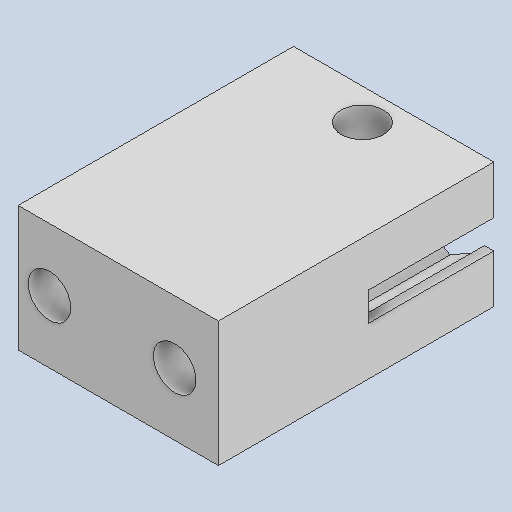
# Autodesk Inventor part: belt_holder
Saved by Autodesk Inventor 2024 (Build 280153000, 153)
## iProperties
Created: 2026-02-15
Part Number: belt_holder
Material: Generic
Document SubType Name: Modeling
Designer: SEMEN
Density: 1 g/cm^3
Appearance: Default
Author: SEMEN
Autodesk Inventor part; units mm, degrees
ref_plane "YZ Plane" through (0, 0, 0) normal (1, 0, 0) x (0, 1, 0)
ref_plane "XZ Plane" through (0, 0, 0) normal (0, 1, 0) x (-1, 0, 0)
sketch "Sketch1" plane through (0, 0, 0) normal (0, 0, 1) x (1, 0, 0)
  circle A0 centre (-12.704, 28.2207) radius 12 projected
  circle A1 centre (-12.704, -22.5861) radius 12 projected
  line L0 (-12.704, 28.2207) -> (-12.704, -22.5861) construction
  line L1 (4.1406, 2.8173) -> (-27.9996, 2.8173) construction
  line L2 (-24.704, -73.8176) -> (-24.704, 176.1824) projected
  line L3 (-5.204, -22.5861) -> (-5.204, 28.2207) projected
  line L4 (-22.204, -2.1827) -> (-6.204, -2.1827)
  line L5 (-6.204, -2.1827) -> (-6.204, 7.8173)
  line L6 (-6.204, 7.8173) -> (-22.204, 7.8173)
  line L7 (-22.204, 7.8173) -> (-22.204, -2.1827)
  circle A2 centre (-9.704, 2.8173) radius 3.5 construction
  circle A3 centre (-19.704, 2.8173) radius 2.5 construction
  point P0 (0, 0)
  point P1 (-12.704, 2.8173)
  dimension "d1" = 10
  dimension "d2" = 5
  dimension "d3" = 7
  dimension "d4" = 5
  dimension "d5" = 10
  constraints: 12 end point, 3 point on line, 2 centre point, 2 coincident, 2 horizontal, 2 parallel, 2 tangent, 1 midpoint, 1 perpendicular, 1 vertical, 1 other
  measures "d1" distance of point (-19.704, 2.817) point (-9.704, 2.817)
  measures "d2" distance from line of L2 point (-19.704, 2.817)
  measures "d3" diameter of A2
  measures "d4" diameter of A3
  measures "d5" distance between parallel lines of L6 L4
ref_plane "Work Plane1" through (-26.704, -73.8176, -12) normal (0, 0, -1) x (0, 1, 0)
extrude "Extrusion1" add sketch "Sketch1" against normal up to surface (12 mm away) contours L7 L6 L5 L4
hole "Hole1" at (-9.704, 2.8173, 0) at (-19.704, 2.8173, 0) direction (0, 0, -1) diameter 3.4 end through all clearance for "Countersunk Head GOST 12876-67" size "M3" standard "GOST"
sketch "Sketch2" plane through (-6.204, 7.8173, -12) normal (0, 0, -1) x (-1, 0, 0)
  line L0 (0, -10) -> (0, 0) projected
  line L1 (16, 0) -> (16, -10) projected
  line L2 (0, -6.15) -> (16, -6.15)
  line L3 (16, -3.85) -> (0, -3.85)
  line L4 (-10.3445, -5) -> (21.7957, -5) construction
  line L5 (16, -10) -> (0, -10) projected
  line L6 (0, 0) -> (16, 0) projected
  point P0 (-6.204, -7.8173)
  dimension "d15" = 2.3
  constraints: 4 end point, 4 point on line, 1 parallel, 1 perpendicular, 1 other
  measures "d15" distance between parallel lines of L3 L2
extrude "Extrusion2" add sketch "Sketch2" along normal blind 10 contours L0 L2 L1 L5 | L0 L6 L1 L3
sketch "Sketch3" plane through (-6.204, 7.8173, -22) normal (0, 0, -1) x (-1, 0, 0)
  line L0 (16.25, -3.4123) -> (16.25, -6.5877)
  line L1 (16.25, -6.5877) -> (13.5, -8.1754)
  line L2 (13.5, -8.1754) -> (10.75, -6.5877)
  line L3 (10.75, -6.5877) -> (10.75, -3.4123)
  line L4 (10.75, -3.4123) -> (13.5, -1.8246)
  line L5 (13.5, -1.8246) -> (16.25, -3.4123)
  line L6 (6.25, -3.4123) -> (6.25, -6.5877)
  line L7 (6.25, -6.5877) -> (3.5, -8.1754)
  line L8 (3.5, -8.1754) -> (0.75, -6.5877)
  line L9 (0.75, -6.5877) -> (0.75, -3.4123)
  line L10 (0.75, -3.4123) -> (3.5, -1.8246)
  line L11 (3.5, -1.8246) -> (6.25, -3.4123)
  line L12 (0, -6.15) -> (0, -3.85) projected
  line L13 (16, -3.85) -> (16, -6.15) projected
  point P0 (-6.204, -7.8173)
  point P1 (3.5, -5)
  point P2 (13.5, -5)
  point P3 (13.5, -5)
  point P4 (3.5, -5)
  dimension "d18" = 5.5
  constraints: 24 end point, 3 parallel, 2 coincident, 26 other
  measures "d18" distance between parallel lines of L0 L3
extrude "Extrusion3" cut sketch "Sketch3" against normal blind 12
sketch "Sketch4" plane through (-22.204, 7.8173, 0) normal (0, 1, 0) x (1, 0, 0)
  line L0 (0, 0) -> (0, 22) projected
  line L1 (16, 0) -> (0, 0) projected
  line L2 (16, 0) -> (16, 22) projected
  line L3 (0, 22) -> (16, 22) projected
  line L4 (16, 0) -> (16, 22) projected
  line L5 (16, 19.5) -> (0, 19.5)
  point P0 (22.204, 0)
  point P1 (8, 19.5)
  dimension "d21" = 2.5
  constraints: 2 end point, 2 point on line, 1 midpoint, 1 perpendicular
  measures "d21" distance between parallel lines of L5 L3
hole "Hole2" at (-14.204, 7.8173, -19.5) direction (0, -1, 0) diameter 3.4 end through all clearance for "Countersunk Head GOST 12876-67" size "M3" standard "GOST"
body "Solid1"
